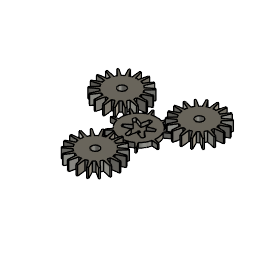
finger_gears (Autodesk Fusion 360 archive; units mm, degrees)
design "finger_gears" references "arm_middle"
part number: 2026-03-18-13-44-59-232
Autodesk Fusion 360 part; units mm, degrees
other "ExternalDerived1"
sketch "Sketch7" plane through (0, 0, 0) normal (0, 0, 1) x (1, 0, 0)
  circle A0 centre (0, 0) radius 19.05
  line L0 (1.2658, -19.0079) -> (0.716, -25.3341)
  line L1 (-1.3142, -19.0046) -> (-0.7583, -25.3302)
  line L2 (0.716, -25.3341) -> (-0.7583, -25.3302)
  line L3 (7.6905, -17.4287) -> (9.3375, -23.5613)
  line L4 (9.3375, -23.5613) -> (7.9509, -24.062)
  line L5 (5.265, -18.308) -> (7.9509, -24.062)
  line L6 (13.1877, -13.7473) -> (16.8329, -18.9468)
  line L7 (16.8329, -18.9468) -> (15.7011, -19.8915)
  line L8 (11.2092, -15.4031) -> (15.7011, -19.8915)
  line L9 (17.0942, -8.4078) -> (22.2979, -12.047)
  line L10 (22.2979, -12.047) -> (21.5575, -13.3218)
  line L11 (15.8014, -10.6405) -> (21.5575, -13.3218)
  line L12 (18.9389, -2.0541) -> (25.0735, -3.6941)
  line L13 (25.0735, -3.6941) -> (24.8137, -5.1453)
  line L14 (18.4877, -4.5944) -> (24.8137, -5.1453)
  line L15 (18.4993, 4.5472) -> (24.8248, 5.1043)
  line L16 (24.8248, 5.1043) -> (25.0771, 3.6518)
  line L17 (18.9441, 2.0059) -> (25.0771, 3.6518)
  line L18 (15.8284, 10.6001) -> (21.582, 13.2871)
  line L19 (21.582, 13.2871) -> (22.3158, 12.0084)
  line L20 (17.1156, 8.3642) -> (22.3158, 12.0084)
  line L21 (11.2484, 15.3745) -> (15.736, 19.8672)
  line L22 (15.736, 19.8672) -> (16.8628, 18.9167)
  line L23 (13.2227, 13.7136) -> (16.8628, 18.9167)
  line L24 (5.3116, 18.2945) -> (7.992, 24.0511)
  line L25 (7.992, 24.0511) -> (9.376, 23.5433)
  line L26 (7.7349, 17.409) -> (9.376, 23.5433)
  line L27 (-1.2658, 19.0079) -> (-0.716, 25.3341)
  line L28 (-0.716, 25.3341) -> (0.7583, 25.3302)
  line L29 (1.3142, 19.0046) -> (0.7583, 25.3302)
  line L30 (-7.6905, 17.4287) -> (-9.3375, 23.5613)
  line L31 (-9.3375, 23.5613) -> (-7.9509, 24.062)
  line L32 (-5.265, 18.308) -> (-7.9509, 24.062)
  line L33 (-13.1877, 13.7473) -> (-16.8329, 18.9468)
  line L34 (-16.8329, 18.9468) -> (-15.7011, 19.8915)
  line L35 (-11.2092, 15.4031) -> (-15.7011, 19.8915)
  line L36 (-17.0942, 8.4078) -> (-22.2979, 12.047)
  line L37 (-22.2979, 12.047) -> (-21.5575, 13.3218)
  line L38 (-15.8014, 10.6405) -> (-21.5575, 13.3218)
  line L39 (-18.9389, 2.0541) -> (-25.0735, 3.6941)
  line L40 (-25.0735, 3.6941) -> (-24.8137, 5.1453)
  line L41 (-18.4877, 4.5944) -> (-24.8137, 5.1453)
  line L42 (-18.4993, -4.5472) -> (-24.8248, -5.1043)
  line L43 (-24.8248, -5.1043) -> (-25.0771, -3.6518)
  line L44 (-18.9441, -2.0059) -> (-25.0771, -3.6518)
  line L45 (-15.8284, -10.6001) -> (-21.582, -13.2871)
  line L46 (-21.582, -13.2871) -> (-22.3158, -12.0084)
  line L47 (-17.1156, -8.3642) -> (-22.3158, -12.0084)
  line L48 (-11.2484, -15.3745) -> (-15.736, -19.8672)
  line L49 (-15.736, -19.8672) -> (-16.8628, -18.9167)
  line L50 (-13.2227, -13.7136) -> (-16.8628, -18.9167)
  line L51 (-5.3116, -18.2945) -> (-7.992, -24.0511)
  line L52 (-7.992, -24.0511) -> (-9.376, -23.5433)
  line L53 (-7.7349, -17.409) -> (-9.376, -23.5433)
  dimension "d61" = 38.1
  dimension "d62" = 6.35
  dimension "d63" = 6.35
  dimension "d65" = 360
  constraint coincident A0.centre origin
  constraint coincident A0 L0.start
  constraint coincident A0 L1.start
  measures "d61" diameter of A0
  measures "d62" distance of L0.start L0.end
  measures "d63" distance of L1.start L1.end
extrude "Extrude7" add sketch "Sketch7" along normal blind 5.08 makes body 1
sketch "Sketch8" plane through (0, 0, 0) normal (0, 0, 1) x (1, 0, 0)
  circle A0 centre (0, 76.2) radius 19.05
  line L0 (1.2378, 57.1903) -> (0.685, 50.8644)
  line L1 (-1.2378, 57.1903) -> (-0.6861, 50.8643)
  line L2 (0.685, 50.8644) -> (-0.6861, 50.8643)
  line L3 (16.8102, 57.2321) -> (15.7599, 56.3507)
  line L4 (13.1674, 62.4333) -> (16.8102, 57.2321)
  line L5 (11.271, 60.842) -> (15.7599, 56.3507)
  line L6 (25.0697, 72.4751) -> (24.8317, 71.1248)
  line L7 (18.9359, 74.118) -> (25.0697, 72.4751)
  line L8 (18.506, 71.68) -> (24.8317, 71.1248)
  line L9 (21.5988, 89.4611) -> (22.2844, 88.2737)
  line L10 (15.844, 86.7769) -> (21.5988, 89.4611)
  line L11 (17.0818, 84.6329) -> (22.2844, 88.2737)
  line L12 (8.0216, 100.242) -> (9.31, 99.7731)
  line L13 (5.3385, 94.4867) -> (8.0216, 100.242)
  line L14 (7.6649, 93.64) -> (9.31, 99.7731)
  line L15 (-9.309, 99.7734) -> (-8.0206, 100.2425)
  line L16 (-7.6649, 93.64) -> (-9.309, 99.7734)
  line L17 (-5.3385, 94.4867) -> (-8.0206, 100.2425)
  line L18 (-22.2838, 88.2746) -> (-21.5983, 89.462)
  line L19 (-17.0818, 84.6329) -> (-22.2838, 88.2746)
  line L20 (-15.844, 86.7769) -> (-21.5983, 89.462)
  line L21 (-24.8318, 71.1259) -> (-25.07, 72.4762)
  line L22 (-18.506, 71.68) -> (-24.8318, 71.1259)
  line L23 (-18.9359, 74.118) -> (-25.07, 72.4762)
  line L24 (-15.7607, 56.3514) -> (-16.8111, 57.2327)
  line L25 (-11.271, 60.842) -> (-15.7607, 56.3514)
  line L26 (-13.1674, 62.4333) -> (-16.8111, 57.2327)
  dimension "d68" = 38.1
  dimension "d69" = 6.35
  dimension "d70" = 6.35
  dimension "d72" = 360
  constraint coincident A0 L0.start
  constraint coincident A0 L1.start
  measures "d68" diameter of A0
  measures "d69" distance of L0.start L0.end
  measures "d70" distance of L1.start L1.end
extrude "Extrude8" add sketch "Sketch8" along normal blind 5.08 separate body makes body 2
move_body "Move21" bodies 2 to x (1, 0, 0) y (0, 1, 0) z (0, 0, 1) at (43.18, -38.1, 0)
move_body "Move22" bodies 2 to x (1, 0, 0) y (0, 1, 0) z (0, 0, 1) at (-5.08, 0, 0)
move_body "Move23" bodies 2 to x (-1, 0, 0) y (0, 1, 0) z (0, 0, -1) at (76.2, 0, 7.62)
move_body "Move25" bodies 1 to x (0.999391, 0.034899, 0) y (-0.034899, 0.999391, 0) z (0, 0, 1) at (1.0397, 64.1158, 0.0186)
move_body "Move27" bodies 1 to x (0.939693, 0.34202, 0) y (-0.34202, 0.939693, 0) z (0, 0, 1) at (18.0551, -3.2469, 0.0176)
sketch "Sketch13" plane through (0, 0, 96.5836) normal (0, 0, 1) x (-1, 0, 0)
  arc A0 (-24.5452, 19.5945) -> (-27.652, 22.2082) centre (-38.2925, 6.4068) ccw
  line L0 (-27.652, 22.2082) -> (-24.9707, 27.9643)
  line L1 (-24.9707, 27.9643) -> (-26.2455, 28.7047)
  line L2 (-26.2455, 28.7047) -> (-29.8847, 23.501)
  arc A1 (-29.8847, 23.501) -> (-33.6981, 24.8945) centre (-38.2925, 6.4068) ccw
  line L3 (-33.6981, 24.8945) -> (-33.1472, 31.2205)
  line L4 (-33.1472, 31.2205) -> (-34.5984, 31.4803)
  line L5 (-34.5984, 31.4803) -> (-36.2383, 25.3457)
  arc A2 (-36.2383, 25.3457) -> (-40.2983, 25.3509) centre (-38.2925, 6.4068) ccw
  line L6 (-40.2983, 25.3509) -> (-41.9443, 31.4839)
  line L7 (-41.9443, 31.4839) -> (-43.3968, 31.2317)
  line L8 (-43.3968, 31.2317) -> (-42.8397, 24.9061)
  arc A3 (-42.8397, 24.9061) -> (-46.6566, 23.5224) centre (-38.2925, 6.4068) ccw
  line L9 (-46.6566, 23.5224) -> (-50.3009, 28.7226)
  line L10 (-50.3009, 28.7226) -> (-51.5796, 27.9888)
  line L11 (-51.5796, 27.9888) -> (-48.8926, 22.2353)
  arc A4 (-48.8926, 22.2353) -> (-52.0061, 19.6295) centre (-38.2925, 6.4068) ccw
  line L12 (-52.0061, 19.6295) -> (-57.2091, 23.2697)
  line L13 (-57.2091, 23.2697) -> (-58.1597, 22.1428)
  line L14 (-58.1597, 22.1428) -> (-53.667, 17.6552)
  arc A5 (-53.667, 17.6552) -> (-55.7015, 14.1417) centre (-38.2925, 6.4068) ccw
  line L15 (-55.7015, 14.1417) -> (-61.8358, 15.7828)
  line L16 (-61.8358, 15.7828) -> (-62.3436, 14.3988)
  line L17 (-62.3436, 14.3988) -> (-56.587, 11.7185)
  arc A6 (-56.587, 11.7185) -> (-57.2971, 7.721) centre (-38.2925, 6.4068) ccw
  line L18 (-57.2971, 7.721) -> (-63.6227, 7.1651)
  line L19 (-63.6227, 7.1651) -> (-63.6265, 5.6908)
  line L20 (-63.6265, 5.6908) -> (-57.3004, 5.141)
  arc A7 (-57.3004, 5.141) -> (-56.6005, 1.1418) centre (-38.2925, 6.4068) ccw
  line L21 (-56.6005, 1.1418) -> (-62.3545, -1.5441)
  line L22 (-62.3545, -1.5441) -> (-61.8538, -2.9307)
  line L23 (-61.8538, -2.9307) -> (-55.7212, -1.2837)
  arc A8 (-55.7212, -1.2837) -> (-53.6956, -4.8024) centre (-38.2925, 6.4068) ccw
  line L24 (-53.6956, -4.8024) -> (-58.184, -9.2943)
  line L25 (-58.184, -9.2943) -> (-57.2393, -10.4261)
  line L26 (-57.2393, -10.4261) -> (-52.0398, -6.7809)
  arc A9 (-52.0398, -6.7809) -> (-48.9329, -9.3946) centre (-38.2925, 6.4068) ccw
  line L27 (-48.9329, -9.3946) -> (-51.6143, -15.1507)
  line L28 (-51.6143, -15.1507) -> (-50.3395, -15.8911)
  line L29 (-50.3395, -15.8911) -> (-46.7002, -10.6874)
  arc A10 (-46.7002, -10.6874) -> (-42.8869, -12.0809) centre (-38.2925, 6.4068) ccw
  line L30 (-42.8869, -12.0809) -> (-43.4378, -18.4069)
  line L31 (-43.4378, -18.4069) -> (-41.9866, -18.6667)
  line L32 (-41.9866, -18.6667) -> (-40.3466, -12.5321)
  arc A11 (-40.3466, -12.5321) -> (-36.2866, -12.5373) centre (-38.2925, 6.4068) ccw
  line L33 (-36.2866, -12.5373) -> (-34.6407, -18.6703)
  line L34 (-34.6407, -18.6703) -> (-33.1882, -18.418)
  line L35 (-33.1882, -18.418) -> (-33.7453, -12.0925)
  arc A12 (-33.7453, -12.0925) -> (-29.9283, -10.7088) centre (-38.2925, 6.4068) ccw
  line L36 (-29.9283, -10.7088) -> (-26.2841, -15.909)
  line L37 (-26.2841, -15.909) -> (-25.0054, -15.1751)
  line L38 (-25.0054, -15.1751) -> (-27.6923, -9.4216)
  arc A13 (-27.6923, -9.4216) -> (-24.5789, -6.8159) centre (-38.2925, 6.4068) ccw
  line L39 (-24.5789, -6.8159) -> (-19.3758, -10.456)
  line L40 (-19.3758, -10.456) -> (-18.4253, -9.3291)
  line L41 (-18.4253, -9.3291) -> (-22.918, -4.8416)
  arc A14 (-22.918, -4.8416) -> (-20.8835, -1.3281) centre (-38.2925, 6.4068) ccw
  line L42 (-20.8835, -1.3281) -> (-14.7492, -2.9692)
  line L43 (-14.7492, -2.9692) -> (-14.2414, -1.5852)
  line L44 (-14.2414, -1.5852) -> (-19.998, 1.0952)
  arc A15 (-19.998, 1.0952) -> (-19.2879, 5.0926) centre (-38.2925, 6.4068) ccw
  line L45 (-19.2879, 5.0926) -> (-12.9623, 5.6485)
  line L46 (-12.9623, 5.6485) -> (-12.9584, 7.1228)
  line L47 (-12.9584, 7.1228) -> (-19.2846, 7.6726)
  arc A16 (-19.2846, 7.6726) -> (-19.9845, 11.6718) centre (-38.2925, 6.4068) ccw
  line L48 (-19.9845, 11.6718) -> (-14.2305, 14.3577)
  line L49 (-14.2305, 14.3577) -> (-14.7311, 15.7444)
  line L50 (-14.7311, 15.7444) -> (-20.8638, 14.0973)
  arc A17 (-20.8638, 14.0973) -> (-22.8893, 17.616) centre (-38.2925, 6.4068) ccw
  line L51 (-22.8893, 17.616) -> (-18.401, 22.1079)
  line L52 (-18.401, 22.1079) -> (-19.3457, 23.2397)
  line L53 (-19.3457, 23.2397) -> (-24.5452, 19.5945)
  circle A18 centre (-38.2925, 6.4068) radius 3.81
  circle A19 centre (-78.74, -57.15) radius 3.81
  circle A20 centre (3.3176, -57.4165) radius 3.81
  dimension "d93" = 7.62
  dimension "d94" = 7.62
  dimension "d95" = 7.62
  constraint concentric A0 A18
  measures "d93" diameter of A18
  measures "d94" diameter of A19
  measures "d95" diameter of A20
move_body "Move30" bodies 2 to x (1, 0, 0) y (0, 1, 0) z (0, 0, 1) at (0, 0, -2.54)
move_body "Move33" bodies 1 to x (0.984808, 0.173648, 0) y (-0.173648, 0.984808, 0) z (0, 0, 1) at (7.6575, -2.701, -0.0412)
move_body "Move35" bodies 1 to x (0.939693, -0.34202, 0) y (0.34202, 0.939693, 0) z (0, 0, 1) at (-15.237, 8.2986, 0.7936)
move_body "Move37" bodies 1 to x (1, 0, 0) y (0, 1, 0) z (0, 0, 1) at (0.2124, 0.0655, 0.0216)
sketch "Sketch14" plane through (0, 0, 0) normal (0, 0, -1) x (1, 0, 0)
  arc A0 (56.606, -33.58) -> (51.2674, -24.3333) centre (38.1, -38.1) ccw
  line L0 (51.2674, -24.3333) -> (54.9111, -19.1327)
  line L1 (54.9111, -19.1327) -> (53.8607, -18.2514)
  line L2 (53.8607, -18.2514) -> (49.371, -22.742)
  arc A1 (49.371, -22.742) -> (39.3378, -19.0903) centre (38.1, -38.1) ccw
  line L3 (39.3378, -19.0903) -> (38.7861, -12.7643)
  line L4 (38.7861, -12.7643) -> (37.415, -12.7644)
  line L5 (37.415, -12.7644) -> (36.8622, -19.0903)
  arc A2 (36.8622, -19.0903) -> (26.829, -22.742) centre (38.1, -38.1) ccw
  line L6 (26.829, -22.742) -> (22.3401, -18.2507)
  line L7 (22.3401, -18.2507) -> (21.2898, -19.1321)
  line L8 (21.2898, -19.1321) -> (24.9326, -24.3333)
  arc A3 (24.9326, -24.3333) -> (19.594, -33.58) centre (38.1, -38.1) ccw
  line L9 (19.594, -33.58) -> (13.2683, -33.0248)
  line L10 (13.2683, -33.0248) -> (13.0303, -34.3751)
  line L11 (13.0303, -34.3751) -> (19.1641, -36.018)
  arc A4 (19.1641, -36.018) -> (21.0182, -46.5329) centre (38.1, -38.1) ccw
  line L12 (21.0182, -46.5329) -> (15.8156, -50.1737)
  line L13 (15.8156, -50.1737) -> (16.5012, -51.3611)
  line L14 (16.5012, -51.3611) -> (22.256, -48.6769)
  arc A5 (22.256, -48.6769) -> (30.4351, -55.54) centre (38.1, -38.1) ccw
  line L15 (30.4351, -55.54) -> (28.79, -61.6731)
  line L16 (28.79, -61.6731) -> (30.0784, -62.142)
  line L17 (30.0784, -62.142) -> (32.7615, -56.3867)
  arc A6 (32.7615, -56.3867) -> (43.4385, -56.3867) centre (38.1, -38.1) ccw
  line L18 (43.4385, -56.3867) -> (46.1206, -62.1425)
  line L19 (46.1206, -62.1425) -> (47.409, -61.6734)
  line L20 (47.409, -61.6734) -> (45.7649, -55.54)
  arc A7 (45.7649, -55.54) -> (53.944, -48.6769) centre (38.1, -38.1) ccw
  line L21 (53.944, -48.6769) -> (59.6983, -51.362)
  line L22 (59.6983, -51.362) -> (60.3838, -50.1746)
  line L23 (60.3838, -50.1746) -> (55.1818, -46.5329)
  arc A8 (55.1818, -46.5329) -> (57.0359, -36.018) centre (38.1, -38.1) ccw
  line L24 (57.0359, -36.018) -> (63.17, -34.3762)
  line L25 (63.17, -34.3762) -> (62.9318, -33.0259)
  line L26 (62.9318, -33.0259) -> (56.606, -33.58)
  circle A9 centre (38.1, -38.1) radius 3.81
  line L27 (41.91, -38.1) -> (39.7016, -50.6065)
  line L28 (34.29, -38.1) -> (36.4922, -50.6076)
  arc A10 (36.4922, -50.6076) -> (39.7016, -50.6065) centre (38.0964, -49.1206) ccw
  line L29 (36.195, -41.3996) -> (48.128, -45.7462)
  arc A11 (48.128, -45.7462) -> (49.7318, -42.9662) centre (47.6423, -43.6134) ccw
  line L30 (40.005, -34.8004) -> (49.7318, -42.9662)
  line L31 (40.005, -41.3996) -> (49.7358, -33.2386)
  arc A12 (49.7358, -33.2386) -> (48.1302, -30.4597) centre (47.6459, -32.5928) ccw
  line L32 (36.195, -34.8004) -> (48.1302, -30.4597)
  line L33 (41.91, -38.1) -> (39.7078, -25.5924)
  arc A13 (39.7078, -25.5924) -> (36.4984, -25.5935) centre (38.1036, -27.0794) ccw
  line L34 (34.29, -38.1) -> (36.4984, -25.5935)
  line L35 (40.005, -34.8004) -> (28.072, -30.4538)
  arc A14 (28.072, -30.4538) -> (26.4682, -33.2338) centre (28.5577, -32.5866) ccw
  line L36 (36.195, -41.3996) -> (26.4682, -33.2338)
  line L37 (36.195, -34.8004) -> (26.4642, -42.9614)
  arc A15 (26.4642, -42.9614) -> (28.0698, -45.7403) centre (28.5541, -43.6072) ccw
  line L38 (40.005, -41.3996) -> (28.0698, -45.7403)
  dimension "d100" = 7.62
  dimension "d101" = 12.7
  dimension "d102" = 12.7
  dimension "d104" = 360
  constraint concentric A0 A9
  constraint coincident A9 L27.start
  constraint coincident A9 L28.start
  measures "d100" diameter of A9
  measures "d101" distance of L27.start L27.end
  measures "d102" distance of L28.start L28.end
extrude "Extrude12" cut sketch "Sketch14" along normal blind 0 and the other way blind 1.27 contours A9 L33 | A9 L27 L30 L31 L33 | A9 L27 | A9 L27 L28 L29 L30 L31 L32 L33 L34 L35 L36 L37 L38 | A9 L30 L33 | A9 L27 L31 | A9 L30 | A9 L30 L32 L33 L35 | L30 L31 A12 L32 L33 | A9 L27 L29 L31 L38 | A9 L31 | L27 L29 A11 L30 L31 | A9 L35 | L32 L33 A13 L34 L35 | A9 L38 | L27 L28 A10 L29 L38 | A9 L32 L35 | A9 L32 L34 L35 L37 | A9 L29 L38 | A9 L28 L29 L36 L38 | A9 L32 | L34 L35 A14 L36 L37 | A9 L29 | L28 L36 L37 A15 L38 | A9 L37 | A9 L34 L37 | A9 L28 L34 L36 L37 | A9 L36 | A9 L28 L36 | A9 L34 | A9 L28 bodies 2
sketch "Sketch15" plane through (0, 0, 1.27) normal (0, 0, -1) x (1, 0, 0)
  arc A0 (28.072, -30.4538) -> (26.4682, -33.2338) centre (28.5577, -32.5866) ccw
  line L0 (26.4682, -33.2338) -> (32.2627, -38.0983)
  line L1 (32.2627, -38.0983) -> (26.4642, -42.9614)
  arc A1 (26.4642, -42.9614) -> (28.0698, -45.7403) centre (28.5541, -43.6072) ccw
  line L2 (28.0698, -45.7403) -> (35.1799, -43.1544)
  line L3 (35.1799, -43.1544) -> (36.4922, -50.6076)
  arc A2 (36.4922, -50.6076) -> (39.7016, -50.6065) centre (38.0964, -49.1206) ccw
  line L4 (39.7016, -50.6065) -> (41.0172, -43.1561)
  line L5 (41.0172, -43.1561) -> (48.128, -45.7462)
  arc A3 (48.128, -45.7462) -> (49.7318, -42.9662) centre (47.6423, -43.6134) ccw
  line L6 (49.7318, -42.9662) -> (43.9373, -38.1017)
  line L7 (43.9373, -38.1017) -> (49.7358, -33.2386)
  arc A4 (49.7358, -33.2386) -> (48.1302, -30.4597) centre (47.6459, -32.5928) ccw
  line L8 (48.1302, -30.4597) -> (41.0201, -33.0456)
  line L9 (41.0201, -33.0456) -> (39.7078, -25.5924)
  arc A5 (39.7078, -25.5924) -> (36.4984, -25.5935) centre (38.1036, -27.0794) ccw
  line L10 (36.4984, -25.5935) -> (35.1828, -33.0439)
  line L11 (35.1828, -33.0439) -> (28.072, -30.4538)
  circle A6 centre (38.1, -38.1) radius 1.27
  dimension "d109" = 2.54
  measures "d109" diameter of A6
extrude "Extrude13" cut sketch "Sketch15" along normal blind 0 and the other way blind 1.27 contours A6 bodies 2
move_body "Move38" bodies 1 to x (1, 0, 0) y (0, 1, 0) z (0, 0, 1) at (0, 0, -0.762)
extrude "Extrude14" cut 1 faces at (31.8375, 42.331, 1.27) along direction (0, 0, -1) blind 0 and the other way blind 2.54 on bodies 2 bodies 2
extrude "Extrude15" cut 1 faces at (37.9453, 37.7608, 2.54) along direction (0, 0, -1) blind 0 and the other way blind 1.27 on bodies 2 bodies 2
move_body "Move39" bodies 2 to x (-1, 0, 0) y (0, 1, 0) z (0, 0, -1) at (76.2003, 0, 5.08)
sketch "Sketch16" plane through (0, 0, 0) normal (0, 0, -1) x (1, 0, 0)
  arc A0 (24.9328, -24.3333) -> (19.5943, -33.58) centre (38.1003, -38.1) ccw
  line L0 (19.5943, -33.58) -> (13.2685, -33.0259)
  line L1 (13.2685, -33.0259) -> (13.0303, -34.3762)
  line L2 (13.0303, -34.3762) -> (19.1644, -36.018)
  arc A1 (19.1644, -36.018) -> (21.0184, -46.5329) centre (38.1003, -38.1) ccw
  line L3 (21.0184, -46.5329) -> (15.8164, -50.1746)
  line L4 (15.8164, -50.1746) -> (16.5019, -51.362)
  line L5 (16.5019, -51.362) -> (22.2563, -48.6769)
  arc A2 (22.2563, -48.6769) -> (30.4354, -55.54) centre (38.1003, -38.1) ccw
  line L6 (30.4354, -55.54) -> (28.7913, -61.6734)
  line L7 (28.7913, -61.6734) -> (30.0797, -62.1425)
  line L8 (30.0797, -62.1425) -> (32.7617, -56.3867)
  arc A3 (32.7617, -56.3867) -> (43.4388, -56.3867) centre (38.1003, -38.1) ccw
  line L9 (43.4388, -56.3867) -> (46.1218, -62.142)
  line L10 (46.1218, -62.142) -> (47.4103, -61.6731)
  line L11 (47.4103, -61.6731) -> (45.7652, -55.54)
  arc A4 (45.7652, -55.54) -> (53.9443, -48.6769) centre (38.1003, -38.1) ccw
  line L12 (53.9443, -48.6769) -> (59.6991, -51.3611)
  line L13 (59.6991, -51.3611) -> (60.3847, -50.1737)
  line L14 (60.3847, -50.1737) -> (55.1821, -46.5329)
  arc A5 (55.1821, -46.5329) -> (57.0362, -36.018) centre (38.1003, -38.1) ccw
  line L15 (57.0362, -36.018) -> (63.17, -34.3751)
  line L16 (63.17, -34.3751) -> (62.932, -33.0248)
  line L17 (62.932, -33.0248) -> (56.6063, -33.58)
  arc A6 (56.6063, -33.58) -> (51.2677, -24.3333) centre (38.1003, -38.1) ccw
  line L18 (51.2677, -24.3333) -> (54.9105, -19.1321)
  line L19 (54.9105, -19.1321) -> (53.8602, -18.2507)
  line L20 (53.8602, -18.2507) -> (49.3713, -22.742)
  arc A7 (49.3713, -22.742) -> (39.3381, -19.0903) centre (38.1003, -38.1) ccw
  line L21 (39.3381, -19.0903) -> (38.7853, -12.7644)
  line L22 (38.7853, -12.7644) -> (37.4142, -12.7643)
  line L23 (37.4142, -12.7643) -> (36.8625, -19.0903)
  arc A8 (36.8625, -19.0903) -> (26.8293, -22.742) centre (38.1003, -38.1) ccw
  line L24 (26.8293, -22.742) -> (22.3396, -18.2514)
  line L25 (22.3396, -18.2514) -> (21.2892, -19.1327)
  line L26 (21.2892, -19.1327) -> (24.9328, -24.3333)
  circle A9 centre (38.1003, -38.1) radius 1.27
  dimension "d122" = 2.54
  constraint concentric A0 A9
  measures "d122" diameter of A9
extrude "Extrude16" cut sketch "Sketch16" against normal blind 24.13 contours A9 bodies 2
move_face "OffsetFaces1" offset -2.54 1 faces at (5.6774, 42.6101, 3.4349) on bodies 1
move_face "OffsetFaces2" offset -2.54 1 faces at (0.5721, 41.2759, 3.4349) on bodies 1
move_face "OffsetFaces3" offset -2.54 1 faces at (-9.0371, 42.6389, 1.7416) on bodies 1
move_face "OffsetFaces4" offset -2.54 1 faces at (11.2507, 46.1752, 3.4349) on bodies 1
move_face "OffsetFaces5" offset -2.54 1 faces at (14.3618, 49.8682, 1.7416) on bodies 1
move_face "OffsetFaces6" offset -2.54 1 faces at (16.9289, 55.9659, 1.7416) on bodies 1
move_face "OffsetFaces7" offset -2.54 2 faces at (17.2822, 62.3521, 1.7416) (16.9406, 64.3752, 1.7416) on bodies 1
move_face "OffsetFaces8" offset -2.54 1 faces at (15.3026, 68.895, 3.4349) on bodies 1
move_face "OffsetFaces9" offset -2.54 1 faces at (11.3054, 74.167, 3.4349) on bodies 1
move_face "OffsetFaces10" offset -2.54 1 faces at (2.7419, 78.7343, 3.4349) on bodies 1
move_face "OffsetFaces11" offset -2.54 1 faces at (-1.1563, 79.2401, 3.4349) on bodies 1
move_face "OffsetFaces12" offset -2.54 1 faces at (-8.9683, 77.7827, 3.4349) on bodies 1
move_face "OffsetFaces13" offset -2.54 1 faces at (-14.5416, 74.2175, 3.4349) on bodies 1
move_face "OffsetFaces14" offset -2.54 1 faces at (-19.1399, 67.7362, 3.4349) on bodies 1
move_face "OffsetFaces15" offset -2.54 1 faces at (-20.5371, 62.6478, 3.4349) on bodies 1
move_face "OffsetFaces16" offset -2.54 1 faces at (-20.5465, 57.819, 1.7416) on bodies 1
move_face "OffsetFaces17" offset -2.54 1 faces at (-18.5935, 51.4978, 1.7416) on bodies 1
move_face "OffsetFaces18" offset -2.54 1 faces at (-12.1086, 44.277, 3.4349) on bodies 1
sketch "Sketch17" plane through (0, 0, 5.1283) normal (0, 0, 1) x (-1, 0, 0)
  arc A0 (8.0504, -44.9794) -> (5.458, -44.1326) centre (1.6455, -60.1964) ccw
  line L0 (5.458, -44.1326) -> (5.9217, -35.2182)
  line L1 (5.9217, -35.2182) -> (4.4623, -35.0092)
  line L2 (4.4623, -35.0092) -> (2.4596, -43.7065)
  arc A1 (2.4596, -43.7065) -> (-0.2661, -43.7974) centre (1.6455, -60.1964) ccw
  line L3 (-0.2661, -43.7974) -> (-2.8793, -35.262)
  line L4 (-2.8793, -35.262) -> (-4.3221, -35.5648)
  line L5 (-4.3221, -35.5648) -> (-3.2294, -44.4225)
  arc A2 (-3.2294, -44.4225) -> (-5.7596, -45.4402) centre (1.6455, -60.1964) ccw
  line L6 (-5.7596, -45.4402) -> (-11.1344, -38.3133)
  line L7 (-11.1344, -38.3133) -> (-12.3867, -39.0913)
  line L8 (-12.3867, -39.0913) -> (-8.3304, -47.041)
  arc A3 (-8.3304, -47.041) -> (-10.3599, -48.8627) centre (1.6455, -60.1964) ccw
  line L9 (-10.3599, -48.8627) -> (-17.8482, -44.004)
  line L10 (-17.8482, -44.004) -> (-18.7588, -45.1634)
  line L11 (-18.7588, -45.1634) -> (-12.2281, -51.2463)
  arc A4 (-12.2281, -51.2463) -> (-13.5122, -53.6523) centre (1.6455, -60.1964) ccw
  line L12 (-13.5122, -53.6523) -> (-22.2107, -51.6477)
  line L13 (-22.2107, -51.6477) -> (-22.6699, -53.0487)
  line L14 (-22.6699, -53.0487) -> (-14.4526, -56.5311)
  arc A5 (-14.4526, -56.5311) -> (-14.8363, -59.2312) centre (1.6455, -60.1964) ccw
  line L15 (-14.8363, -59.2312) -> (-23.6958, -60.3226)
  line L16 (-23.6958, -60.3226) -> (-23.6482, -61.7961)
  line L17 (-23.6482, -61.7961) -> (-14.7353, -62.258)
  arc A6 (-14.7353, -62.258) -> (-14.1724, -64.9265) centre (1.6455, -60.1964) ccw
  line L18 (-14.1724, -64.9265) -> (-22.1244, -68.9822)
  line L19 (-22.1244, -68.9822) -> (-21.5757, -70.3505)
  line L20 (-21.5757, -70.3505) -> (-13.0423, -67.7363)
  arc A7 (-13.0423, -67.7363) -> (-11.6007, -70.0513) centre (1.6455, -60.1964) ccw
  line L21 (-11.6007, -70.0513) -> (-17.686, -76.5821)
  line L22 (-17.686, -76.5821) -> (-16.7023, -77.6802)
  line L23 (-16.7023, -77.6802) -> (-9.5777, -72.3051)
  arc A8 (-9.5777, -72.3051) -> (-7.4313, -73.9874) centre (1.6455, -60.1964) ccw
  line L24 (-7.4313, -73.9874) -> (-10.9159, -82.2057)
  line L25 (-10.9159, -82.2057) -> (-9.616, -82.9012)
  line L26 (-9.616, -82.9012) -> (-4.7595, -75.4134)
  arc A9 (-4.7595, -75.4134) -> (-2.1671, -76.2602) centre (1.6455, -60.1964) ccw
  line L27 (-2.1671, -76.2602) -> (-2.6307, -85.1746)
  line L28 (-2.6307, -85.1746) -> (-1.1714, -85.3835)
  line L29 (-1.1714, -85.3835) -> (0.8313, -76.6863)
  arc A10 (0.8313, -76.6863) -> (3.557, -76.5954) centre (1.6455, -60.1964) ccw
  line L30 (3.557, -76.5954) -> (6.1702, -85.1308)
  line L31 (6.1702, -85.1308) -> (7.613, -84.828)
  line L32 (7.613, -84.828) -> (6.5203, -75.9703)
  arc A11 (6.5203, -75.9703) -> (9.0505, -74.9526) centre (1.6455, -60.1964) ccw
  line L33 (9.0505, -74.9526) -> (14.4254, -82.0795)
  line L34 (14.4254, -82.0795) -> (15.6776, -81.3015)
  line L35 (15.6776, -81.3015) -> (11.6213, -73.3517)
  arc A12 (11.6213, -73.3517) -> (13.6508, -71.53) centre (1.6455, -60.1964) ccw
  line L36 (13.6508, -71.53) -> (21.1391, -76.3888)
  line L37 (21.1391, -76.3888) -> (22.0498, -75.2294)
  line L38 (22.0498, -75.2294) -> (15.5191, -69.1464)
  arc A13 (15.5191, -69.1464) -> (16.8031, -66.7404) centre (1.6455, -60.1964) ccw
  line L39 (16.8031, -66.7404) -> (25.5016, -68.745)
  line L40 (25.5016, -68.745) -> (25.9608, -67.3441)
  line L41 (25.9608, -67.3441) -> (17.7435, -63.8616)
  arc A14 (17.7435, -63.8616) -> (18.1272, -61.1616) centre (1.6455, -60.1964) ccw
  line L42 (18.1272, -61.1616) -> (26.9867, -60.0702)
  line L43 (26.9867, -60.0702) -> (26.9391, -58.5967)
  line L44 (26.9391, -58.5967) -> (18.0262, -58.1347)
  arc A15 (18.0262, -58.1347) -> (17.4634, -55.4663) centre (1.6455, -60.1964) ccw
  line L45 (17.4634, -55.4663) -> (25.4153, -51.4106)
  line L46 (25.4153, -51.4106) -> (24.8666, -50.0422)
  line L47 (24.8666, -50.0422) -> (16.3332, -52.6565)
  arc A16 (16.3332, -52.6565) -> (14.8916, -50.3415) centre (1.6455, -60.1964) ccw
  line L48 (14.8916, -50.3415) -> (20.9769, -43.8107)
  line L49 (20.9769, -43.8107) -> (19.9933, -42.7125)
  line L50 (19.9933, -42.7125) -> (12.8687, -48.0877)
  arc A17 (12.8687, -48.0877) -> (10.7222, -46.4053) centre (1.6455, -60.1964) ccw
  line L51 (10.7222, -46.4053) -> (14.2068, -38.1871)
  line L52 (14.2068, -38.1871) -> (12.9069, -37.4916)
  line L53 (12.9069, -37.4916) -> (8.0504, -44.9794)
  circle A18 centre (1.6455, -60.1964) radius 4.064
  dimension "d143" = 8.128
  constraint concentric A0 A18
  measures "d143" diameter of A18
extrude "Extrude17" cut sketch "Sketch17" against normal blind 12.7 contours A18 bodies 1
extrude "Extrude18" add 1 faces at (10.0676, 56.394, 5.1283) along direction (0, 0, 1) blind 2.54 on bodies 1 bodies 1
extrude "Extrude19" add 1 faces at (10.0676, 56.394, 7.6683) along direction (0, 0, 1) blind 5.08 on bodies 1 bodies 1
extrude "Extrude20" cut 1 faces at (10.0676, 56.394, 12.7483) along direction (0, 0, -1) blind 2.54 on bodies 1 bodies 1
copy_body "CopyPasteBodies5" bodies 1 makes body 3
move_body "Move42" bodies 3 to x (1, 0, 0) y (0, 1, 0) z (0, 0, 1) at (68.58, 12.7, 0)
copy_body "CopyPasteBodies6" bodies 1 makes body 4
move_body "Move43" bodies 4 to x (1, 0, 0) y (0, 1, 0) z (0, 0, 1) at (40.64, -68.58, 0)
